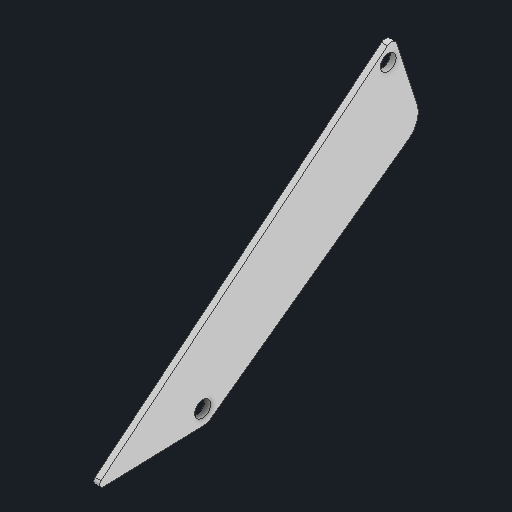
# Autodesk Inventor part: ramp_v3
Saved by Autodesk Inventor 2025 (Build 290162000, 162)
## iProperties
Created: 2024-10-13
Part Number: ramp_v3
Material: Generic
Document SubType Name: Modeling
Designer: Averey Ku
Density: 1 g/cm^3
Appearance: Default
Author: Averey Ku
Autodesk Inventor part; units mm, degrees
ref_plane "YZ Plane" through (0, 0, 0) normal (1, 0, 0) x (0, 1, 0)
ref_plane "XZ Plane" through (0, 0, 0) normal (0, 1, 0) x (-1, 0, 0)
ref_plane "XY Plane" through (0, 0, 0) normal (0, 0, 1) x (1, 0, 0)
sketch "Sketch1" plane through (0, 0, 0) normal (1, 0, 0) x (0, 1, 0)
  arc A0 (-26.0803, 50.1701) -> (-27.9475, 49.6154) centre (-26.9315, 49.6154) ccw
  circle A1 centre (-23.185, 23.3761) radius 2.1209
  circle A2 centre (16.5025, -27.4239) radius 2.1209 construction
  line L0 (-26.2163, 50.337) -> (35.6741, -25.6248)
  arc A3 (11.3565, -31.1442) -> (18.4564, -33.4658) centre (16.5025, -27.4239) ccw
  arc A4 (-27.1519, 23.2564) -> (-26.1603, 20.7496) centre (-23.185, 23.3761) ccw
  line L1 (-26.1603, 20.7496) -> (11.3565, -31.1442)
  line L2 (18.4564, -33.4658) -> (34.9319, -28.138)
  arc A5 (34.9319, -28.138) -> (35.6741, -25.6248) centre (34.4434, -26.6275) ccw
  circle A6 centre (31.7468, -25.8311) radius 2.0828
  line L3 (-27.1519, 23.2564) -> (-27.9475, 49.6154)
  point P0 (0, 0)
  point P1 (-27.9475, 67.8261)
  dimension "d1" = 12.7
  dimension "d2" = 4.1656
  constraints: 10 point on circle, 8 end point, 7 centre point, 5 tangent, 2 coincident, 1 point on line, 5 other
  measures "d1" diameter of A3
  measures "d2" diameter of A6
extrude "Extrusion1" add sketch "Sketch1" along normal blind 1.5875 contours L0 A5 L2 A3 L1 A4 L3 A0
body "Solid1"
